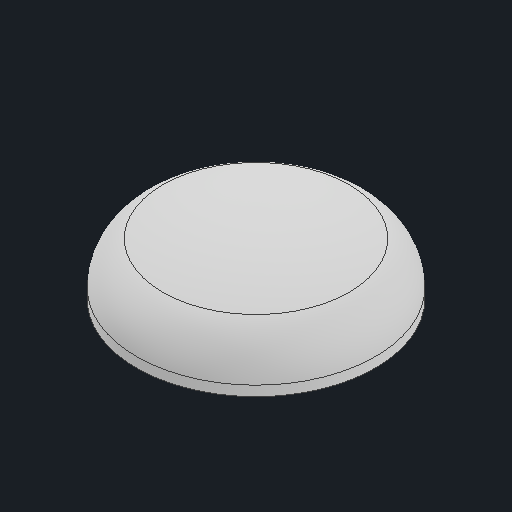
# Autodesk Inventor part: Fuel Cap Outlet
Saved by Autodesk Inventor 2026 (Build 300175050, 175E)
## iProperties
Created: 2026-03-18
Part Number: Fuel Cap Outlet
Material: Generic
Document SubType Name: Modeling
Designer: jackr
Density: 1 g/cm^3
Appearance: Default
Inner_D: 5.450 in
Thickness: 0.550 in
Skirt_Length: 0.500 in
Knuckle: 1.853 in
Crown: 9.810 in
Thickness_Top: 0.550 in
Outside_Knuckle: 2.403 in
Tank_Outer_Diameter: 12.000 in
Tank_Inner_Diameter: 10.510 in
Outlet_Cap_Wall_Thickness: 0.550 in
Outlet_Cap_Knuckle_Radius: 1.853 in
Outlet_Cap_Crown_Radius: 9.810 in
Outlet_Cap_Skirt_Length: 0.500 in
Author: jackr
Autodesk Inventor part; units mm, degrees
ref_plane "YZ Plane" through (0, 0, 0) normal (1, 0, 0) x (0, 1, 0)
ref_plane "XZ Plane" through (0, 0, 0) normal (0, 1, 0) x (-1, 0, 0)
ref_plane "XY Plane" through (0, 0, 0) normal (0, 0, 1) x (1, 0, 0)
sketch "Sketch1" plane through (0, 0, 0) normal (0, 0, 1) x (1, 0, 0)
  arc A0 (0, 81.5958) -> (-112.6403, 54.6826) centre (0, -167.5782) ccw
  arc A1 (-112.6403, 54.6826) -> (-138.43, 12.7) centre (-91.3638, 12.7) ccw
  line L0 (-138.43, 12.7) -> (-138.43, 0)
  line L1 (-138.43, 0) -> (-152.4, 0)
  line L2 (-152.4, 0) -> (-152.4, 12.7)
  line L3 (0, 95.5658) -> (0, 81.5958)
  line L4 (0, -221.6084) -> (0, 156.6029) projected
  line L5 (-182.0818, 12.7) -> (-119.4588, 12.7) construction
  line L6 (-218.4982, 0) -> (36.4164, 0) projected
  arc A2 (-118.9555, 67.1437) -> (-152.4, 12.7) centre (-91.3638, 12.7) ccw
  arc A3 (0, 95.5658) -> (-118.9555, 67.1437) centre (0, -167.5782) ccw
  point P0 (-145.415, 0)
  dimension "Inner_D" = 138.43
  dimension "Thickness" = 13.97
  dimension "Skirt_Length" = 12.7
  dimension "Knuckle" = 47.0662
  dimension "Crown" = 249.174
  dimension "Thickness_Top" = 13.97
  dimension "Outside_Knuckle" = 61.0362
  constraints: 10 end point, 8 point on circle, 4 centre point, 4 tangent, 2 collinear, 2 line through centre, 2 perpendicular, 2 point on line, 2 vertical, 1 horizontal, 1 midpoint
  measures "Inner_D" distance between parallel lines of L4 L0
  measures "Thickness" distance of L0.end L1.end
  measures "Skirt_Length" distance from line of point (-145.415, 0) L5
  measures "Knuckle" radius of A1
  measures "Crown" radius of A0
  measures "Thickness_Top" distance of L3.start L3.end
  measures "Outside_Knuckle" radius of A2
revolve "Revolution2" add sketch "Sketch1" angle 360 about axis through (0, -10, 0) along (0, 1, 0) contours A0 A1 L0 L1 L2 A2 A3 L3
equation "\"Thickness\" = Outlet_Cap_Wall_Thickness"
equation "\"Skirt_Length\" = Outlet_Cap_Skirt_Length"
equation "\"Knuckle\" = Outlet_Cap_Knuckle_Radius"
equation "\"Outlet_Cap_Wall_Thickness\" = 13.97"
equation "\"Outlet_Cap_Knuckle_Radius\" = 47.0662"
equation "\"Outlet_Cap_Skirt_Length\" = 12.7"
body "Solid2"
